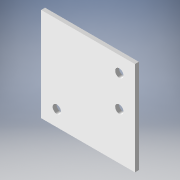
# Autodesk Inventor part: 15102898-16-P-0220
Saved by Autodesk Inventor 2017 (Build 210142000, 142)
## iProperties
Created: 2016-10-16
Part Number: 15102898-16-P-0220
Material: Generic
Document SubType Name: Modeling
Designer: gus
Density: 1 g/cm^3
Appearance: Default
Author: gus
Autodesk Inventor part; units mm, degrees
ref_plane "YZ Plane" through (0, 0, 0) normal (1, 0, 0) x (0, 1, 0)
ref_plane "XZ Plane" through (0, 0, 0) normal (0, 1, 0) x (-1, 0, 0)
ref_plane "XY Plane" through (0, 0, 0) normal (0, 0, 1) x (1, 0, 0)
sketch "Sketch1" plane through (0, 0, 0) normal (0, 0, 1) x (1, 0, 0)
  line L0 (0, 0) -> (-76.2, 0)
  line L1 (-76.2, 0) -> (-76.2, 76.2)
  line L2 (-76.2, 76.2) -> (0, 76.2)
  line L3 (0, 76.2) -> (0, 0)
  circle A0 centre (-12.7, 63.5) radius 3.3734
  circle A1 centre (-12.7, 38.1) radius 3.3734
  circle A2 centre (-63.5, 12.7) radius 3.3734
  dimension "d0" = 76.2
  dimension "d1" = 76.2
  dimension "d2" = 6.7469
  dimension "d3" = 12.7
  dimension "d4" = 12.7
  dimension "d5" = 38.1
  dimension "d6" = 12.7
  dimension "d7" = 12.7
  dimension "d8" = 12.7
  constraints: 8 end point, 3 centre point, 2 equal radius, 2 parallel, 1 horizontal, 1 perpendicular
  measures "d0" distance of L1.end L2.end
  measures "d1" distance of L0.end L1.end
  measures "d2" diameter of A0
  measures "d3" distance from line of L3 A0.centre
  measures "d4" distance from line of L3 A1.centre
  measures "d5" distance from line of L0 A1.centre
  measures "d6" distance from line of L2 A0.centre
  measures "d7" distance from line of L0 A2.centre
  measures "d8" distance from line of L1 A2.centre
extrude "Extrusion1" add sketch "Sketch1" along normal blind 3.175
body "Solid1"
